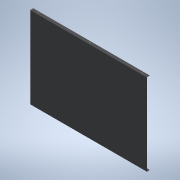
# Autodesk Inventor part: SP41V1 Cubre Base
Saved by Autodesk Inventor 2021.2 (Build 252289000, 289)
## iProperties
Created: 2026-08-25
Part Number: SP41V1 Cubre Base
Material: Generic
Document SubType Name: Sheet Metal
Designer: nelso
Density: 1 g/cm^3
Sheet Metal Rule: Default_mm
Appearance: Gray
Author: nelso
Autodesk Inventor part; units mm, degrees
ref_plane "YZ Plane" through (0, 0, 0) normal (1, 0, 0) x (0, 1, 0)
ref_plane "XZ Plane" through (0, 0, 0) normal (0, 1, 0) x (-1, 0, 0)
ref_plane "XY Plane" through (0, 0, 0) normal (0, 0, 1) x (1, 0, 0)
sketch "Sketch1" plane through (0, 0, 0) normal (0, 1, 0) x (-1, 0, 0)
  line L0 (381.5, 268.3) -> (-381.5, 268.3)
  line L1 (-381.5, 268.3) -> (-381.5, -268.3)
  line L2 (-381.5, -268.3) -> (381.5, -268.3)
  line L3 (381.5, -268.3) -> (381.5, 268.3)
  line L4 (381.5, 268.3) -> (-381.5, -268.3) construction
  line L5 (-381.5, 268.3) -> (381.5, -268.3) construction
  point P0 (0, 0)
  dimension "d0" = 763
  dimension "d1" = 536.6
  measures "d0" distance of L2.end L1.end
  measures "d1" distance of L1.end L0.end
extrude "Plate1" add sketch "Sketch1" along normal blind 0.9
sketch "Sketch2" plane through (381.5, 0, 267.4) normal (0, 0, 1) x (1, 0, 0)
  line L0 (-763, 0) -> (0, 0)
  line L1 (0, 0) -> (0, 20)
  line L2 (0, 20) -> (-763, 20)
  line L3 (-763, 20) -> (-763, 0)
  constraints: 6 end point, 1 horizontal, 1 perpendicular, 1 vertical
edge flange "Flange1" height 20 angle 90 thickness 0.9 bend radius 1.008 thickness toward (0, 0, 1) relief straight relief width 0.9 relief depth 0.45 corner gap 1.008 corner form 0 edges at (0, 0.9, 268.3) (0, 0.9, -268.3) wall of the first edge with corners at (-381.5, 0, 267.4) (381.5, 0, 267.4) (381.5, 20, 267.4) (-381.5, 20, 267.4)
bend "Bend1"
corner "Corner1"
sketch "Sketch3" plane through (-381.5, 20, 268.3) normal (0, 0, 1) x (1, 0, 0)
  circle A0 centre (723.3, -11) radius 1.7
  circle A1 centre (381.5, -11) radius 1.7
  circle A2 centre (39.7, -11) radius 1.7
  line L0 (0, 0) -> (763, 0) projected
  point P0 (381.5, -20)
  dimension "d20" = 11
  dimension "d21" = 11
  dimension "d22" = 11
  constraints: 3 centre point, 3 coincident
  measures "d20" distance from line of L0 point (39.7, -11)
  measures "d21" distance from line of L0 A1.centre
  measures "d22" distance from line of L0 A0.centre
hole "Hole1" at (-341.8, 9, 268.3) at (0, 9, 268.3) at (341.8, 9, 268.3) direction (0, 0, -1) diameter 6 end through all
equation "\"d18\" = Thickness"
equation "\"d2\" = Thickness"
equation "\"d3\" = BendReliefWidth"
equation "\"d4\" = BendReliefDepth"
equation "\"d5\" = MinimumRemnant"
equation "\"d6\" = TransitionRadius"
equation "\"d9\" = BendRadius"
equation "\"d10\" = CornerReliefSize"
equation "\"d11\" = GapSize"
equation "\"d12\" = JacobiRadiusSize"
equation "\"BendReliefWidth\" = Thickness"
equation "\"BendReliefDepth\" = 0.5 * Thickness"
equation "\"CornerReliefSize\" = 4 * Thickness"
equation "\"MinimumRemnant\" = 2 * Thickness"
equation "\"TransitionRadius\" = BendRadius"
equation "\"JacobiRadiusSize\" = BendRadius"
equation "\"GapSize\" = Thickness"
equation "\"Thickness\" = 0.9"
equation "\"BendRadius\" = 1.008"
body "Solid1"
